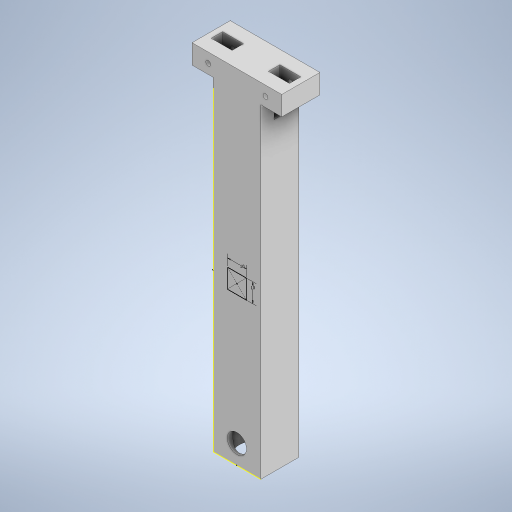
# Autodesk Inventor part: Tensile_test_bottom_adapter_blocked
Saved by Autodesk Inventor 2024 (Build 280153000, 153)
## iProperties
Created: 2023-09-15
Part Number: Tensile_test_bottom_adapter_blocked
Material: 일반
Document SubType Name: Modeling
Designer: jsw
Density: 1 g/cm^3
Appearance: 기본값
Author: jsw
Autodesk Inventor part; units mm, degrees
ref_plane "YZ Plane" through (0, 0, 0) normal (1, 0, 0) x (0, 1, 0)
sketch "스케치1" plane through (0, 0, 0) normal (0, 1, 0) x (-1, 0, 0)
  line L0 (-12.5, 10) -> (12.5, 10)
  line L1 (12.5, 10) -> (12.5, -10)
  line L2 (12.5, -10) -> (-12.5, -10)
  line L3 (-12.5, -10) -> (-12.5, 10)
  line L4 (-12.5, 10) -> (12.5, -10) construction
  line L5 (12.5, 10) -> (-12.5, -10) construction
  circle A0 centre (0, 0) radius 8.75
  dimension "d0" = 25
  dimension "d1" = 20
  dimension "d2" = 17.5
  constraints: 12 end point, 2 midpoint, 2 parallel, 1 centre point, 1 coincident, 1 horizontal, 1 perpendicular
  measures "d0" distance of L1.end L2.end
  measures "d1" distance of L0.end L1.end
  measures "d2" diameter of A0
extrude "돌출1" add sketch "스케치1" along normal blind 20
sketch "스케치2" plane through (12.5, 0, -10) normal (0, 0, -1) x (-1, 0, 0)
  circle A0 centre (12.5, 10) radius 5
  line L0 (0, 0) -> (25, 0) projected
  point P0 (12.5, 0)
  point P1 (12.5, 0)
  point P2 (12.5, 0)
  dimension "d5" = 10
  dimension "d6" = 10
  constraints: 2 midpoint, 1 centre point, 1 vertical alignment
  measures "d5" diameter of A0
  measures "d6" distance of point (12.5, 0) A0.centre
extrude "돌출2" cut sketch "스케치2" against normal up to surface (20 mm away)
sketch "스케치3" plane through (0, 20, 0) normal (0, 1, 0) x (1, 0, 0)
  line L0 (12.5, 10) -> (-12.5, 10) projected
  line L1 (-12.5, 10) -> (-12.5, -10) projected
  line L2 (-12.5, -10) -> (12.5, -10) projected
  line L3 (12.5, -10) -> (12.5, 10) projected
  circle A0 centre (0, 0) radius 8.75 projected
extrude "돌출3" add sketch "스케치3" along normal blind 160 contours L3 L2 L1 L0 | A0
sketch "스케치21" plane through (-12.5, 0, 10) normal (0, 0, 1) x (1, 0, 0)
  line L0 (25, 180) -> (0, 180) projected
  line L1 (25, 0) -> (25, 180) projected
  line L2 (0, 180) -> (25, 180)
  line L3 (25, 180) -> (25, 165)
  line L4 (25, 165) -> (0, 165)
  line L5 (0, 165) -> (0, 180)
  point P0 (12.5, 0)
  dimension "d153" = 15
  constraints: 8 end point, 2 parallel, 1 horizontal, 1 perpendicular, 1 point on line
  measures "d153" distance of L2.end L3.end
extrude "돌출8" cut sketch "스케치21" against normal blind 0.5
ref_plane "작업 평면1" through (12.5, 0, 0) normal (0, 0, -1) x (-1, 0, 0)
mirror "미러1" about plane through (12.5, 0, 0) normal (0, 0, -1) of "돌출8"
sketch "스케치23" plane through (0, 180, 0) normal (0, 1, 0) x (1, 0, 0)
  circle A0 centre (0, 0) radius 4.5
  line L0 (-2.5981, -4.5) -> (-5.1962, 0)
  line L1 (-5.1962, 0) -> (-2.5981, 4.5)
  line L2 (-2.5981, 4.5) -> (2.5981, 4.5)
  line L3 (2.5981, 4.5) -> (5.1962, 0)
  line L4 (5.1962, 0) -> (2.5981, -4.5)
  line L5 (2.5981, -4.5) -> (-2.5981, -4.5)
  dimension "d162" = 9
  constraints: 12 end point, 2 coincident, 1 centre point, 1 horizontal, 1 tangent, 13 other
  measures "d162" diameter of A0
extrude "돌출10" cut sketch "스케치23" against normal blind 8
sketch "스케치25" plane through (0, 172, 0) normal (0, 1, 0) x (1, 0, 0)
  line L0 (2.0207, 3.5) -> (4.0415, 0)
  line L1 (4.0415, 0) -> (2.0207, -3.5)
  line L2 (2.0207, -3.5) -> (-2.0207, -3.5)
  line L3 (-2.0207, -3.5) -> (-4.0415, 0)
  line L4 (-4.0415, 0) -> (-2.0207, 3.5)
  line L5 (-2.0207, 3.5) -> (2.0207, 3.5)
  line L6 (-5.1962, 0) -> (-2.5981, 4.5) projected
  line L7 (2.5981, -4.5) -> (-2.5981, -4.5) projected
  line L8 (5.1962, 0) -> (2.5981, -4.5) projected
  line L9 (2.5981, 4.5) -> (5.1962, 0) projected
  line L10 (-2.5981, 4.5) -> (2.5981, 4.5) projected
  line L11 (-5.1962, 0) -> (-2.5981, 4.5) projected
  line L12 (-2.5981, -4.5) -> (-5.1962, 0) projected
  point P0 (0, 0)
  point P1 (0, 0)
  dimension "d166" = 1
  constraints: 12 end point, 1 coincident, 1 horizontal, 13 other
  measures "d166" distance between parallel lines of L4 L6
extrude "돌출11" add sketch "스케치25" along normal blind 4.5
sketch "스케치26" plane through (0, 180, 0) normal (0, 1, 0) x (1, 0, 0)
  line L0 (23.5, 10) -> (-23.5, 10)
  line L1 (-23.5, 10) -> (-23.5, -10)
  line L2 (-23.5, -10) -> (23.5, -10)
  line L3 (23.5, -10) -> (23.5, 10)
  line L4 (23.5, 10) -> (-23.5, -10) construction
  line L5 (-23.5, 10) -> (23.5, -10) construction
  line L6 (-9.5, 3) -> (-20.5, 3)
  line L7 (-20.5, 3) -> (-20.5, -3)
  line L8 (-20.5, -3) -> (-9.5, -3)
  line L9 (-9.5, -3) -> (-9.5, 3)
  line L10 (-9.5, 3) -> (-20.5, -3) construction
  line L11 (-20.5, 3) -> (-9.5, -3) construction
  line L12 (-12.5, -9.5) -> (12.5, -9.5) projected
  line L13 (0, -9.5) -> (0, 10)
  line L14 (-5, 10) -> (5, 10) projected
  line L15 (23.5, 10) -> (23.5, -10)
  line L16 (9.5, 3) -> (20.5, 3)
  line L17 (20.5, 3) -> (20.5, -3)
  line L18 (20.5, -3) -> (9.5, -3)
  line L19 (9.5, -3) -> (9.5, 3)
  point P0 (0, 0)
  point P1 (-15, 0)
  dimension "d169" = 15
  dimension "d170" = 11
  dimension "d172" = 3
  dimension "d173" = 6
  dimension "d174" = 7
  constraints: 36 end point, 6 midpoint, 4 parallel, 4 symmetric about line, 2 horizontal, 2 perpendicular, 1 horizontal alignment
  measures "d169" distance from line of point (-15, 0) L13
  measures "d170" distance of L6.start L6.end
  measures "d172" distance between parallel lines of L7 L1
  measures "d173" distance of L6.end L7.end
  measures "d174" distance between parallel lines of L2 L8
extrude "돌출12" add sketch "스케치26" against normal blind 10.16
sketch "스케치27" plane through (0, 180, 0) normal (0, 1, 0) x (1, 0, 0)
  line L0 (-9.5, 3) -> (-12.5, 3)
  line L1 (-12.5, 3) -> (-12.5, -3)
  line L2 (-12.5, -3) -> (-9.5, -3)
  line L3 (-9.5, -3) -> (-9.5, 3)
  line L4 (-9.5, 3) -> (-12.5, -3) construction
  line L5 (-12.5, 3) -> (-9.5, -3) construction
  line L6 (0, 0) -> (0, 9.5)
  line L7 (12.5, 9.5) -> (-12.5, 9.5) projected
  line L8 (9.5, 3) -> (12.5, 3)
  line L9 (12.5, 3) -> (12.5, -3)
  line L10 (12.5, -3) -> (9.5, -3)
  line L11 (9.5, -3) -> (9.5, 3)
  line L12 (9.5, 3) -> (12.5, -3) construction
  line L13 (12.5, 3) -> (9.5, -3) construction
  point P0 (-11, 0)
  point P1 (11, 0)
  dimension "d177" = 9.5
  dimension "d178" = 3
  dimension "d179" = 6
  constraints: 26 end point, 5 symmetric about line, 3 midpoint, 2 parallel, 1 horizontal, 1 horizontal alignment, 1 perpendicular
  measures "d177" distance from line of L6.start L3
  measures "d178" distance of L0.start L0.end
  measures "d179" distance of L0.end L1.end
extrude "돌출13" cut sketch "스케치27" against normal blind 20.32
sketch "스케치28" plane through (-12.5, 0, 10) normal (0, 0, 1) x (1, 0, 0)
  line L0 (7.5, 87.5) -> (17.5, 87.5)
  line L1 (17.5, 87.5) -> (17.5, 77.5)
  line L2 (17.5, 77.5) -> (7.5, 77.5)
  line L3 (7.5, 77.5) -> (7.5, 87.5)
  line L4 (7.5, 87.5) -> (17.5, 77.5) construction
  line L5 (17.5, 87.5) -> (7.5, 77.5) construction
  line L6 (0, 0) -> (25, 0) projected
  line L7 (0, 0) -> (0, 165) projected
  point P0 (12.5, 0)
  point P1 (12.5, 82.5)
  point P2 (12.5, 0)
  point P3 (0, 82.5)
  dimension "d184" = 10
  dimension "d185" = 10
  constraints: 12 end point, 4 midpoint, 2 parallel, 1 horizontal, 1 horizontal alignment, 1 perpendicular, 1 vertical alignment
  measures "d184" distance of L0.end L1.end
  measures "d185" distance of L0.start L0.end
sketch "스케치29" plane through (12.5, 165, -9.5) normal (0, 0, -1) x (-1, 0, 0)
  line L0 (0, 0) -> (25, 0) projected
  line L1 (25, 4.84) -> (25, 0) projected
  line L2 (0, 0) -> (0, 4.84) projected
  line L3 (25, 4.84) -> (0, 4.84) projected
  point P0 (12.5, -165)
extrude "돌출14" add sketch "스케치29" along normal blind 0.5
ref_plane "작업 평면2" through (12.5, 0, 0) normal (0, 0, -1) x (-1, 0, 0)
mirror "미러2" about plane through (12.5, 0, 0) normal (0, 0, -1) of "돌출14"
sketch "스케치30" plane through (-12.5, 0, 10) normal (0, 0, 1) x (1, 0, 0)
  circle A0 centre (27.5, 174.92) radius 1.25
  line L0 (36, 180) -> (36, 169.84) projected
  line L1 (0, 0) -> (0, 169.84) projected
  line L2 (25, 0) -> (25, 169.84) projected
  line L3 (0, 169.84) -> (25, 169.84)
  line L4 (25, 169.84) -> (12.5, 169.84)
  line L5 (-11, 180) -> (36, 180) projected
  line L6 (12.5, 180) -> (12.5, 169.84)
  circle A1 centre (-2.5, 174.92) radius 1.25
  point P0 (12.5, 0)
  point P1 (36, 174.92)
  dimension "d186" = 2.5
  dimension "d187" = 8.5
  constraints: 6 end point, 3 midpoint, 2 centre point, 1 horizontal, 1 horizontal alignment, 1 perpendicular, 1 symmetric about line, 1 other
  measures "d186" diameter of A0
  measures "d187" distance from line of A0.centre L0
extrude "돌출15" cut sketch "스케치30" against normal up to surface (20 mm away)
equation "\"d34\" = 55deg"
equation "\"d54\" = 55deg"
equation "\"d74\" = 55deg"
equation "\"d94\" = 55deg"
equation "\"d116\" = 55deg"
equation "\"d136\" = 55deg"
